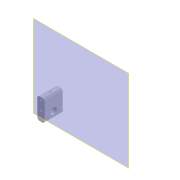
# Autodesk Inventor part: 40_Cube_XY_Table_Aliexpress_naked_illuminationarm_block_12V_13.5mm_Lamp
Saved by Autodesk Inventor 2022 (Build 260153000, 153)
## iProperties
Created: 2022-12-09
Part Number: 40_Cube_XY_Table_Aliexpress_naked_illuminationarm_block_12V_13.5mm_Lamp
Material: Generisch
Document SubType Name: Modeling
Designer: diederichbenedict
Density: 1 g/cm^3
Appearance: Vorgabe
Author: diederichbenedict
Autodesk Inventor part; units mm, degrees
ref_plane "YZ Plane" through (0, 0, 0) normal (1, 0, 0) x (0, 1, 0)
ref_plane "XZ Plane" through (0, 0, 0) normal (0, 1, 0) x (-1, 0, 0)
ref_plane "Arbeitsebene4" through (119.9133, 130.103, 38) normal (0, 0, -1) x (0.0001363, -1, 0)
sketch "Skizze4" plane through (119.9133, 130.103, 38) normal (0, 0, -1) x (0.0001363, -1, 0)
  arc A0 (-32.8643, -10.3064) -> (-24.3863, -15.0021) centre (-24.3869, -5.0021) ccw projected
  line L0 (-24.3863, -15.0021) -> (12.0741, -14.9996) projected
  line L1 (12.0741, -14.9996) -> (12.0705, 15.0004) projected
  line L2 (12.0705, 15.0004) -> (-10.9295, 14.9976) projected
  line L3 (-10.9295, 14.9976) -> (-13.6953, 14.9974) projected
  arc A1 (-23.696, 24.9968) -> (-13.6953, 14.9974) centre (-13.696, 24.9974) ccw projected
  line L4 (-23.696, 24.9968) -> (-23.7027, 123.1353) projected
  arc A2 (-20.7742, 130.2066) -> (-23.7027, 123.1353) centre (-13.7027, 123.136) ccw projected
  line L5 (-20.7742, 130.2066) -> (-0.8384, 150.1451) projected
  arc A3 (6.2324, 153.0745) -> (-0.8384, 150.1451) centre (6.2331, 143.0745) ccw projected
  line L6 (6.2324, 153.0745) -> (109.3857, 153.0815) projected
  line L7 (109.3857, 153.0815) -> (109.3847, 168.0815) projected
  line L8 (109.3847, 168.0815) -> (-7.648, 168.0735) projected
  arc A4 (-7.648, 168.0735) -> (-13.9491, 165.8381) centre (-7.6473, 158.0735) ccw projected
  line L9 (-13.9491, 165.8381) -> (-45.0051, 140.6329) projected
  arc A5 (-45.0051, 140.6329) -> (-48.7033, 132.8676) centre (-38.7033, 132.8683) ccw projected
  line L10 (-48.7033, 132.8676) -> (-48.6955, 17.8654) projected
  arc A6 (-48.6955, 17.8654) -> (-47.1728, 12.5618) centre (-38.6955, 17.866) ccw projected
  line L11 (-47.1728, 12.5618) -> (-32.8643, -10.3064) projected
  circle A7 centre (8.0736, -11.0001) radius 1.4 projected
  circle A8 centre (8.071, 10.9999) radius 1.4 projected
  circle A9 centre (8.0722, 1.0566) radius 1.4 projected
  circle A10 centre (3.7693, -11.0006) radius 1.4 projected
  circle A11 centre (-6.6177, 10.9981) radius 1.4 projected
  circle A12 centre (-1.4242, -0.0012) radius 1.4 projected
  circle A13 centre (1.2315, 10.9991) radius 1.4 projected
  circle A14 centre (-40.6775, 25.6744) radius 1.5 projected
  circle A15 centre (-40.6796, 55.6744) radius 1.5 projected
  circle A16 centre (-30.6796, 55.6751) radius 1.5 projected
  circle A17 centre (-30.6775, 25.6751) radius 1.5 projected
  circle A18 centre (55.2542, 160.5778) radius 1.5 projected
  circle A19 centre (104.3852, 160.5812) radius 1.5 projected
  circle A20 centre (84.3852, 160.5798) radius 1.5 projected
  circle A21 centre (35.2542, 160.5765) radius 1.5 projected
  line L12 (99.7638, 71.6425) -> (99.7669, 45.3925)
  line L13 (125.7638, 71.6456) -> (125.7669, 45.3956)
  line L14 (79.3852, 168.0795) -> (124.3852, 168.0795)
  line L15 (124.3852, 168.0795) -> (124.3852, 153.2355)
  line L16 (124.3852, 153.2355) -> (79.3852, 153.2355)
  line L17 (79.3852, 153.2355) -> (79.3852, 168.0795)
  point P0 (130.0867, 119.931)
  dimension "d21" = 5
  dimension "d22" = 20
  constraints: 12 end point, 2 parallel, 1 horizontal, 1 perpendicular, 1 point on line, 6 other
  measures "d21" distance from line of L17 A20.centre
  measures "d22" distance from line of L15 A19.centre
ref_plane "Arbeitsebene5" through (-48.1749, 20.6944, 0) normal (0, 0, 1) x (1, 0.0001363, 0)
extrude "Extrusion3" add sketch "Skizze4" along normal up to surface (38 mm away) contours L8 L7 L16 L17 | L14 L15 L16 L7
chamfer "Fase2" distance 3 angle 45 4 edges at (-48.1492, 5.6949, 19) (-33.3052, 5.6969, 19) (-48.1554, 50.6949, 19) (-33.3114, 50.6969, 19)
sketch "Skizze5" plane through (-48.155, 47.6949, 0) normal (-1, -0.0001363, 0) x (0, 0, 1)
  ellipse E0 centre (19, -30.3773) end of major axis (11.8839, -30.3773) minor radius 7.1161 projected
  circle A0 centre (19, -30.3773) radius 6.75
  point P0 (0, -47.7015)
  dimension "d28" = 13.5
  constraints: 1 centre point, 1 coincident, 1 other
  measures "d28" diameter of A0
extrude "Extrusion4" cut sketch "Skizze5" against normal through all contours A0
sketch "Skizze6" plane through (-36.3052, 5.6965, 0) normal (0.0001363, -1, 0) x (1, 0.0001363, 0)
  circle A0 centre (-4.3457, 19) radius 1.4
  point P0 (36.3045, 0)
  dimension "d31" = 2.8
  constraints: 1 centre point, 1 other
  measures "d31" diameter of A0
extrude "Extrusion5" cut sketch "Skizze6" against normal through all
